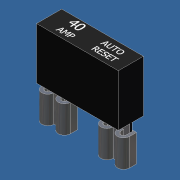
# Autodesk Inventor part: Big CB in Holder
Saved by Autodesk Inventor 2012 (Build 160160000, 160)
## iProperties
Company: Team 801
Created: 2007-09-01
Part Number: Big CB in Holder
Document SubType Name: Modeling
Designer: Jeffrey M
Manufacturer: Standard
Standards Organization: Custom
Mass: 5.35109 g
Surface Area: 29.8147 cm^2
Volume: 5.35109 cm^3
Density: 1 g/cm^3
Catalog Web Link: www.team801.org
Material: Default
PartAngTol0: 0.50 deg
PartAngTol1: 0.50 deg
PartAngTol2: 0.50 deg
PartLinTol0: 0.01 in
PartLinTol1: 0.01 in
PartLinTol2: 0.01 in
PartLinTol3: 0.005 in
PartAngTol3: 0deg30'
Author: Jeffrey M
Autodesk Inventor part; units mm, degrees
ref_plane "YZ Plane (RIGHT)" through (0, 0, 0) normal (1, 0, 0) x (0, 1, 0)
ref_plane "XZ Plane (TOP)" through (0, 0, 0) normal (0, 1, 0) x (-1, 0, 0)
ref_plane "XY Plane (FRONT)" through (0, 0, 0) normal (0, 0, 1) x (1, 0, 0)
sketch "Sketch2" plane through (0, 0, 0) normal (0, 1, 0) x (-1, 0, 0)
  line L0 (-23.1648, 0) -> (17.3736, 0) construction
  line L1 (0, -5.334) -> (0, 7.112) construction
  line L2 (-14.478, 4.445) -> (14.478, 4.445)
  line L3 (14.478, 4.445) -> (14.478, -4.445)
  line L4 (14.478, -4.445) -> (-14.478, -4.445)
  line L5 (-14.478, -4.445) -> (-14.478, 4.445)
  dimension "d0" = 28.956
  dimension "d1" = 8.89
  constraints: 8 end point, 2 parallel, 1 horizontal, 1 perpendicular, 2 other
  measures "d0" distance of L2.start L2.end
  measures "d1" distance of L4.end L2.start
extrude "Extrusion1" add sketch "Sketch2" along normal blind 18.288
sketch "Sketch3" plane through (0, 0, 0) normal (0, -1, 0) x (1, 0, 0)
  line L0 (-14.478, 4.445) -> (-14.478, -4.445) construction
  line L1 (0, 7.112) -> (0, -5.334) construction
  line L2 (-17.3736, 0) -> (23.1648, 0) construction
  line L3 (-14.478, 0.4064) -> (-6.477, 0.4064)
  line L4 (-6.477, 0.4064) -> (-6.477, -0.4064)
  line L5 (-6.477, -0.4064) -> (-14.478, -0.4064)
  line L6 (-14.478, -0.4064) -> (-14.478, 0.4064)
  line L7 (14.478, 0.4064) -> (6.477, 0.4064)
  line L8 (6.477, 0.4064) -> (6.477, -0.4064)
  line L9 (6.477, -0.4064) -> (14.478, -0.4064)
  line L10 (14.478, -0.4064) -> (14.478, 0.4064)
  dimension "d4" = 0.8128
  dimension "d5" = 8.001
  constraints: 16 end point, 4 symmetric about line, 2 parallel, 1 horizontal, 1 perpendicular, 1 point on line, 1 other
  measures "d4" distance between parallel lines of L3 L5
  measures "d5" distance of L4.end L5.end
extrude "Extrusion2" add sketch "Sketch3" along normal blind 12.446
sketch "Sketch4" plane through (0, -12.446, 0) normal (0, -1, 0) x (1, 0, 0)
  line L0 (-6.477, 0.4064) -> (-6.477, -0.4064) projected
  line L1 (-14.478, 0.4064) -> (-6.477, 0.4064) projected
  line L2 (-14.478, -0.4064) -> (-14.478, 0.4064) projected
  line L3 (-6.477, -0.4064) -> (-14.478, -0.4064) projected
  line L4 (-15.5575, -0.9652) -> (-5.3975, -0.9652)
  line L5 (-5.3975, -0.9652) -> (-5.3975, 1.524)
  arc A0 (-5.3975, 1.524) -> (-9.7155, 1.524) centre (-7.5565, 1.524) ccw
  line L6 (-9.7155, 1.524) -> (-11.2395, 1.524)
  arc A1 (-11.2395, 1.524) -> (-15.5575, 1.524) centre (-13.3985, 1.524) ccw
  line L7 (-15.5575, 1.524) -> (-15.5575, -0.9652)
  line L8 (-10.4775, 0.4064) -> (-10.4775, 5.8427) construction
  line L9 (-14.478, 0.4064) -> (-14.478, 1.524)
  arc A2 (-12.319, 1.524) -> (-14.478, 1.524) centre (-13.3985, 1.524) ccw
  line L10 (-12.319, 1.524) -> (-12.319, 0.4064)
  line L11 (-6.477, 0.4064) -> (-6.477, 1.524)
  arc A3 (-6.477, 1.524) -> (-8.636, 1.524) centre (-7.5565, 1.524) ccw
  line L12 (-8.636, 1.524) -> (-8.636, 0.4064)
  point P0 (0, 0)
  dimension "d8" = 0.5588
  dimension "d9" = 10.16
  dimension "d10" = 4.6482
  dimension "d11" = 1.524
  constraints: 18 end point, 8 point on circle, 7 parallel, 6 tangent, 4 centre point, 3 perpendicular, 3 point on line, 2 coincident, 1 midpoint, 1 other
  measures "d8" distance between parallel lines of L4 L3
  measures "d9" distance of L4.start L4.end
  measures "d11" distance of L6.start L6.end
extrude "Extrusion3" add sketch "Sketch4" against normal blind 9.652
mirror "Mirror1" about plane through (0, 0, 0) normal (1, 0, 0) of "Extrusion3"
sketch "Sketch5" plane through (0, 18.288, 0) normal (0, 1, 0) x (1, 0, 0)
  line L0 (-9.1661, 3.7805) -> (-3.0835, 3.7805) construction
  line L1 (-3.0835, 3.7805) -> (-3.0835, -3.7805) construction
  line L2 (-3.0835, -3.7805) -> (-9.1661, -3.7805) construction
  line L3 (-9.1661, -3.7805) -> (-9.1661, 3.7805) construction
  line L4 (2.9146, 2.7245) -> (10.9734, 2.7245) construction
  line L5 (10.9734, 2.7245) -> (10.9734, -2.7322) construction
  line L6 (10.9734, -2.7322) -> (2.9146, -2.7322) construction
  line L7 (2.9146, -2.7322) -> (2.9146, 2.7245) construction
  line L8 (-6.9826, 1.718) -> (-7.3457, 1.718)
  line L9 (-7.3457, 1.718) -> (-7.3457, 0.6707)
  line L10 (-7.3457, 0.6707) -> (-7.7384, 0.6707)
  line L11 (-7.7384, 0.6707) -> (-7.7384, 1.718)
  line L12 (-7.7384, 1.718) -> (-9.0846, 1.718)
  line L13 (-9.0846, 1.718) -> (-9.0846, 2.1478)
  line L14 (-9.0846, 2.1478) -> (-7.7211, 3.7187)
  line L15 (-7.7211, 3.7187) -> (-7.3457, 3.7187)
  line L16 (-7.3457, 3.7187) -> (-7.3457, 2.0465)
  line L17 (-7.3457, 2.0465) -> (-6.9826, 2.0465)
  line L18 (-6.9826, 2.0465) -> (-6.9826, 1.718)
  line L19 (-7.7384, 2.0465) -> (-7.7384, 3.2371)
  line L20 (-7.7384, 3.2371) -> (-8.7635, 2.0465)
  line L21 (-8.7635, 2.0465) -> (-7.7384, 2.0465)
  spline S0 degree 2 poles (-4.7596, 2.1947) (-4.7596, 1.3747) (-5.2363, 0.6065) (-5.7328, 0.6065) knots 0 0 0 1 2 2 2
  spline S1 degree 2 poles (-5.7328, 0.6065) (-6.2367, 0.6065) (-6.7084, 1.3895) (-6.7084, 2.1923) knots 0 0 0 1 2 2 2
  spline S2 degree 2 poles (-6.7084, 2.1923) (-6.7084, 3.0172) (-6.2317, 3.7805) (-5.7328, 3.7805) knots 0 0 0 1 2 2 2
  spline S3 degree 2 poles (-5.7328, 3.7805) (-5.2314, 3.7805) (-4.7596, 2.9901) (-4.7596, 2.1947) knots 0 0 0 1 2 2 2
  spline S4 degree 2 poles (-5.2832, 1.266) (-5.2239, 1.4167) (-5.1745, 1.881) (-5.1745, 2.1947) knots 0 0 0 1 2 2 2
  spline S5 degree 2 poles (-5.1745, 2.1947) (-5.1745, 2.5084) (-5.2239, 2.9703) (-5.2857, 3.1259) knots 0 0 0 1 2 2 2
  spline S6 degree 2 poles (-5.2857, 3.1259) (-5.3474, 3.2815) (-5.5623, 3.4421) (-5.7328, 3.4421) knots 0 0 0 1 2 2 2
  spline S7 degree 2 poles (-5.7328, 3.4421) (-5.9032, 3.4421) (-6.123, 3.2815) (-6.1873, 3.121) knots 0 0 0 1 2 2 2
  spline S8 degree 2 poles (-6.1873, 3.121) (-6.249, 2.9654) (-6.2935, 2.4911) (-6.2935, 2.1923) knots 0 0 0 1 2 2 2
  spline S9 degree 2 poles (-6.2935, 2.1923) (-6.2935, 1.8712) (-6.2539, 1.4414) (-6.1897, 1.2734) knots 0 0 0 1 2 2 2
  spline S10 degree 2 poles (-6.1897, 1.2734) (-6.1304, 1.1153) (-5.9106, 0.9449) (-5.7328, 0.9449) knots 0 0 0 1 2 2 2
  spline S11 degree 2 poles (-5.7328, 0.9449) (-5.5648, 0.9449) (-5.345, 1.1055) (-5.2832, 1.266) knots 0 0 0 1 2 2 2
  line L22 (-9.1793, -3.067) -> (-8.4942, -1.035)
  line L23 (-8.4942, -1.035) -> (-8.1616, -1.035)
  line L24 (-8.1616, -1.035) -> (-7.4766, -3.067)
  line L25 (-7.4766, -3.067) -> (-7.7615, -3.067)
  line L26 (-7.7615, -3.067) -> (-7.9459, -2.4989)
  line L27 (-7.9459, -2.4989) -> (-8.7215, -2.4989)
  line L28 (-8.7215, -2.4989) -> (-8.9059, -3.067)
  line L29 (-8.9059, -3.067) -> (-9.1793, -3.067)
  line L30 (-8.02, -2.2683) -> (-8.3345, -1.3116)
  line L31 (-8.3345, -1.3116) -> (-8.6474, -2.2683)
  line L32 (-8.6474, -2.2683) -> (-8.02, -2.2683)
  line L33 (-5.5418, -3.067) -> (-5.8118, -3.067)
  line L34 (-5.8118, -3.067) -> (-5.8118, -1.3166)
  line L35 (-5.8118, -1.3166) -> (-6.342, -2.5071)
  line L36 (-6.342, -2.5071) -> (-6.5067, -2.5071)
  line L37 (-6.5067, -2.5071) -> (-7.032, -1.3166)
  line L38 (-7.032, -1.3166) -> (-7.032, -3.067)
  line L39 (-7.032, -3.067) -> (-7.2839, -3.067)
  line L40 (-7.2839, -3.067) -> (-7.2839, -1.035)
  line L41 (-7.2839, -1.035) -> (-6.9151, -1.035)
  line L42 (-6.9151, -1.035) -> (-6.4079, -2.1662)
  line L43 (-6.4079, -2.1662) -> (-5.9172, -1.035)
  line L44 (-5.9172, -1.035) -> (-5.5418, -1.035)
  line L45 (-5.5418, -1.035) -> (-5.5418, -3.067)
  spline S12 degree 2 poles (-3.8457, -1.6475) (-3.8457, -1.7793) (-3.9395, -2.0164) (-4.0235, -2.0987) knots 0 0 0 1 2 2 2
  spline S13 degree 2 poles (-4.0235, -2.0987) (-4.1289, -2.2025) (-4.4138, -2.3095) (-4.6311, -2.3095) knots 0 0 0 1 2 2 2
  line L46 (-4.6311, -2.3095) -> (-4.86, -2.3095)
  line L47 (-4.86, -2.3095) -> (-4.86, -3.067)
  line L48 (-4.86, -3.067) -> (-5.1301, -3.067)
  line L49 (-5.1301, -3.067) -> (-5.1301, -1.035)
  line L50 (-5.1301, -1.035) -> (-4.6196, -1.035)
  spline S14 degree 2 poles (-4.6196, -1.035) (-4.4385, -1.035) (-4.1849, -1.0942) (-4.0877, -1.1618) knots 0 0 0 1 2 2 2
  spline S15 degree 2 poles (-4.0877, -1.1618) (-3.9741, -1.2392) (-3.8457, -1.4779) (-3.8457, -1.6475) knots 0 0 0 1 2 2 2
  spline S16 degree 2 poles (-4.1273, -1.6558) (-4.1273, -1.5504) (-4.1997, -1.3956) (-4.2738, -1.3462) knots 0 0 0 1 2 2 2
  spline S17 degree 2 poles (-4.2738, -1.3462) (-4.338, -1.3034) (-4.5093, -1.2688) (-4.6361, -1.2688) knots 0 0 0 1 2 2 2
  line L51 (-4.6361, -1.2688) -> (-4.86, -1.2688)
  line L52 (-4.86, -1.2688) -> (-4.86, -2.079)
  line L53 (-4.86, -2.079) -> (-4.6756, -2.079)
  spline S18 degree 2 poles (-4.6756, -2.079) (-4.5109, -2.079) (-4.3084, -2.0263) (-4.2425, -1.9571) knots 0 0 0 1 2 2 2
  spline S19 degree 2 poles (-4.2425, -1.9571) (-4.1816, -1.8962) (-4.1273, -1.7529) (-4.1273, -1.6558) knots 0 0 0 1 2 2 2
  line L54 (2.9014, 0.6497) -> (3.5864, 2.6817)
  line L55 (3.5864, 2.6817) -> (3.919, 2.6817)
  line L56 (3.919, 2.6817) -> (4.6041, 0.6497)
  line L57 (4.6041, 0.6497) -> (4.3192, 0.6497)
  line L58 (4.3192, 0.6497) -> (4.1348, 1.2178)
  line L59 (4.1348, 1.2178) -> (3.3592, 1.2178)
  line L60 (3.3592, 1.2178) -> (3.1747, 0.6497)
  line L61 (3.1747, 0.6497) -> (2.9014, 0.6497)
  line L62 (4.0607, 1.4483) -> (3.7461, 2.405)
  line L63 (3.7461, 2.405) -> (3.4333, 1.4483)
  line L64 (3.4333, 1.4483) -> (4.0607, 1.4483)
  spline S20 degree 2 poles (5.5064, 0.6069) (5.3269, 0.6069) (5.0602, 0.7007) (4.9663, 0.7946) knots 0 0 0 1 2 2 2
  spline S21 degree 2 poles (4.9663, 0.7946) (4.8593, 0.9) (4.772, 1.1964) (4.772, 1.4137) knots 0 0 0 1 2 2 2
  line L65 (4.772, 1.4137) -> (4.772, 2.6817)
  line L66 (4.772, 2.6817) -> (5.0421, 2.6817)
  line L67 (5.0421, 2.6817) -> (5.0421, 1.4137)
  spline S22 degree 2 poles (5.0421, 1.4137) (5.0421, 1.2721) (5.0783, 1.0811) (5.1293, 1.0037) knots 0 0 0 1 2 2 2
  spline S23 degree 2 poles (5.1293, 1.0037) (5.1837, 0.9214) (5.3714, 0.8374) (5.5064, 0.8374) knots 0 0 0 1 2 2 2
  spline S24 degree 2 poles (5.5064, 0.8374) (5.6332, 0.8374) (5.8308, 0.9214) (5.8852, 1.0037) knots 0 0 0 1 2 2 2
  spline S25 degree 2 poles (5.8852, 1.0037) (5.9362, 1.0811) (5.9724, 1.2705) (5.9724, 1.4071) knots 0 0 0 1 2 2 2
  line L68 (5.9724, 1.4071) -> (5.9724, 2.6817)
  line L69 (5.9724, 2.6817) -> (6.2425, 2.6817)
  line L70 (6.2425, 2.6817) -> (6.2425, 1.4137)
  spline S26 degree 2 poles (6.2425, 1.4137) (6.2425, 1.2013) (6.1569, 0.8983) (6.0482, 0.7946) knots 0 0 0 1 2 2 2
  spline S27 degree 2 poles (6.0482, 0.7946) (5.951, 0.6991) (5.6942, 0.6069) (5.5064, 0.6069) knots 0 0 0 1 2 2 2
  line L71 (7.1037, 0.6497) -> (7.1037, 2.4413)
  line L72 (7.1037, 2.4413) -> (6.422, 2.4413)
  line L73 (6.422, 2.4413) -> (6.422, 2.6817)
  line L74 (6.422, 2.6817) -> (8.0555, 2.6817)
  line L75 (8.0555, 2.6817) -> (8.0555, 2.4413)
  line L76 (8.0555, 2.4413) -> (7.3738, 2.4413)
  line L77 (7.3738, 2.4413) -> (7.3738, 0.6497)
  line L78 (7.3738, 0.6497) -> (7.1037, 0.6497)
  spline S28 degree 2 poles (9.6989, 2.4495) (9.8141, 2.3145) (9.9426, 1.9193) (9.9426, 1.6657) knots 0 0 0 1 2 2 2
  spline S29 degree 2 poles (9.9426, 1.6657) (9.9426, 1.4187) (9.8174, 1.0185) (9.6989, 0.8835) knots 0 0 0 1 2 2 2
  spline S30 degree 2 poles (9.6989, 0.8835) (9.5737, 0.7419) (9.2427, 0.6069) (9.0435, 0.6069) knots 0 0 0 1 2 2 2
  spline S31 degree 2 poles (9.0435, 0.6069) (8.8377, 0.6069) (8.5083, 0.7468) (8.3881, 0.8835) knots 0 0 0 1 2 2 2
  spline S32 degree 2 poles (8.3881, 0.8835) (8.2712, 1.0185) (8.1461, 1.4154) (8.1461, 1.6657) knots 0 0 0 1 2 2 2
  spline S33 degree 2 poles (8.1461, 1.6657) (8.1461, 1.9209) (8.2729, 2.3095) (8.3898, 2.4495) knots 0 0 0 1 2 2 2
  spline S34 degree 2 poles (8.3898, 2.4495) (8.5083, 2.5845) (8.8393, 2.7245) (9.0435, 2.7245) knots 0 0 0 1 2 2 2
  spline S35 degree 2 poles (9.0435, 2.7245) (9.251, 2.7245) (9.5836, 2.5796) (9.6989, 2.4495) knots 0 0 0 1 2 2 2
  spline S36 degree 2 poles (9.661, 1.6657) (9.661, 1.8666) (9.5737, 2.1778) (9.4947, 2.2799) knots 0 0 0 1 2 2 2
  spline S37 degree 2 poles (9.4947, 2.2799) (9.414, 2.3853) (9.1868, 2.4907) (9.0451, 2.4907) knots 0 0 0 1 2 2 2
  spline S38 degree 2 poles (9.0451, 2.4907) (8.8986, 2.4907) (8.6779, 2.3886) (8.594, 2.2799) knots 0 0 0 1 2 2 2
  spline S39 degree 2 poles (8.594, 2.2799) (8.5133, 2.1761) (8.4276, 1.8633) (8.4276, 1.6657) knots 0 0 0 1 2 2 2
  spline S40 degree 2 poles (8.4276, 1.6657) (8.4276, 1.2655) (8.7636, 0.8407) (9.0451, 0.8407) knots 0 0 0 1 2 2 2
  spline S41 degree 2 poles (9.0451, 0.8407) (9.3267, 0.8407) (9.661, 1.2655) (9.661, 1.6657) knots 0 0 0 1 2 2 2
  line L79 (4.693, -2.696) -> (4.3422, -2.696)
  line L80 (4.3422, -2.696) -> (3.7, -1.8874)
  line L81 (3.7, -1.8874) -> (3.3905, -1.8874)
  line L82 (3.3905, -1.8874) -> (3.3905, -2.696)
  line L83 (3.3905, -2.696) -> (3.1204, -2.696)
  line L84 (3.1204, -2.696) -> (3.1204, -0.664)
  line L85 (3.1204, -0.664) -> (3.644, -0.664)
  spline S42 degree 2 poles (3.644, -0.664) (3.8186, -0.664) (4.0541, -0.7018) (4.1611, -0.771) knots 0 0 0 1 2 2 2
  spline S43 degree 2 poles (4.1611, -0.771) (4.2681, -0.8402) (4.3916, -1.0559) (4.3916, -1.2156) knots 0 0 0 1 2 2 2
  spline S44 degree 2 poles (4.3916, -1.2156) (4.3916, -1.4379) (4.1644, -1.7392) (3.9701, -1.8117) knots 0 0 0 1 2 2 2
  line L86 (3.9701, -1.8117) -> (4.693, -2.696)
  spline S45 degree 2 poles (4.1101, -1.237) (4.1101, -1.1481) (4.0475, -1.0114) (3.9816, -0.967) knots 0 0 0 1 2 2 2
  spline S46 degree 2 poles (3.9816, -0.967) (3.924, -0.9291) (3.7708, -0.8978) (3.6589, -0.8978) knots 0 0 0 1 2 2 2
  line L87 (3.6589, -0.8978) -> (3.3905, -0.8978)
  line L88 (3.3905, -0.8978) -> (3.3905, -1.6619)
  line L89 (3.3905, -1.6619) -> (3.6276, -1.6619)
  spline S47 degree 2 poles (3.6276, -1.6619) (3.7445, -1.6619) (3.9306, -1.6207) (3.9948, -1.5565) knots 0 0 0 1 2 2 2
  spline S48 degree 2 poles (3.9948, -1.5565) (4.0541, -1.5005) (4.1101, -1.3424) (4.1101, -1.237) knots 0 0 0 1 2 2 2
  line L90 (4.8543, -2.696) -> (4.8543, -0.664)
  line L91 (4.8543, -0.664) -> (6.1256, -0.664)
  line L92 (6.1256, -0.664) -> (6.1256, -0.9044)
  line L93 (6.1256, -0.9044) -> (5.1244, -0.9044)
  line L94 (5.1244, -0.9044) -> (5.1244, -1.461)
  line L95 (5.1244, -1.461) -> (6.0581, -1.461)
  line L96 (6.0581, -1.461) -> (6.0581, -1.7014)
  line L97 (6.0581, -1.7014) -> (5.1244, -1.7014)
  line L98 (5.1244, -1.7014) -> (5.1244, -2.4555)
  line L99 (5.1244, -2.4555) -> (6.1256, -2.4555)
  line L100 (6.1256, -2.4555) -> (6.1256, -2.696)
  line L101 (6.1256, -2.696) -> (4.8543, -2.696)
  spline S49 degree 2 poles (6.9884, -2.7322) (6.7678, -2.7322) (6.4582, -2.64) (6.3215, -2.5741) knots 0 0 0 1 2 2 2
  line L102 (6.3215, -2.5741) -> (6.3215, -2.2349)
  line L103 (6.3215, -2.2349) -> (6.3413, -2.2349)
  spline S50 degree 2 poles (6.3413, -2.2349) (6.4747, -2.36) (6.8122, -2.4984) (6.9687, -2.4984) knots 0 0 0 1 2 2 2
  spline S51 degree 2 poles (6.9687, -2.4984) (7.1926, -2.4984) (7.4215, -2.3123) (7.4215, -2.1591) knots 0 0 0 1 2 2 2
  spline S52 degree 2 poles (7.4215, -2.1591) (7.4215, -2.0373) (7.3013, -1.8858) (7.1712, -1.8479) knots 0 0 0 1 2 2 2
  spline S53 degree 2 poles (7.1712, -1.8479) (7.0774, -1.8216) (6.9209, -1.7854) (6.804, -1.7557) knots 0 0 0 1 2 2 2
  spline S54 degree 2 poles (6.804, -1.7557) (6.6986, -1.7277) (6.5323, -1.6437) (6.4681, -1.5762) knots 0 0 0 1 2 2 2
  spline S55 degree 2 poles (6.4681, -1.5762) (6.4055, -1.5087) (6.3364, -1.3276) (6.3364, -1.209) knots 0 0 0 1 2 2 2
  spline S56 degree 2 poles (6.3364, -1.209) (6.3364, -0.962) (6.7217, -0.6277) (7.0197, -0.6277) knots 0 0 0 1 2 2 2
  spline S57 degree 2 poles (7.0197, -0.6277) (7.191, -0.6277) (7.494, -0.6953) (7.6241, -0.7595) knots 0 0 0 1 2 2 2
  line L104 (7.6241, -0.7595) -> (7.6241, -1.0822)
  line L105 (7.6241, -1.0822) -> (7.6043, -1.0822)
  spline S58 degree 2 poles (7.6043, -1.0822) (7.5071, -0.9933) (7.2042, -0.8616) (7.0378, -0.8616) knots 0 0 0 1 2 2 2
  spline S59 degree 2 poles (7.0378, -0.8616) (6.8501, -0.8616) (6.6179, -1.0378) (6.6179, -1.181) knots 0 0 0 1 2 2 2
  spline S60 degree 2 poles (6.6179, -1.181) (6.6179, -1.3095) (6.7546, -1.4626) (6.8831, -1.4972) knots 0 0 0 1 2 2 2
  spline S61 degree 2 poles (6.8831, -1.4972) (6.9687, -1.5202) (7.2173, -1.5795) (7.2997, -1.6042) knots 0 0 0 1 2 2 2
  spline S62 degree 2 poles (7.2997, -1.6042) (7.5088, -1.6684) (7.7031, -1.927) (7.7031, -2.1163) knots 0 0 0 1 2 2 2
  spline S63 degree 2 poles (7.7031, -2.1163) (7.7031, -2.2365) (7.6059, -2.4671) (7.5187, -2.5478) knots 0 0 0 1 2 2 2
  spline S64 degree 2 poles (7.5187, -2.5478) (7.4215, -2.6367) (7.1745, -2.7322) (6.9884, -2.7322) knots 0 0 0 1 2 2 2
  line L106 (7.9781, -2.696) -> (7.9781, -0.664)
  line L107 (7.9781, -0.664) -> (9.2493, -0.664)
  line L108 (9.2493, -0.664) -> (9.2493, -0.9044)
  line L109 (9.2493, -0.9044) -> (8.2482, -0.9044)
  line L110 (8.2482, -0.9044) -> (8.2482, -1.461)
  line L111 (8.2482, -1.461) -> (9.1818, -1.461)
  line L112 (9.1818, -1.461) -> (9.1818, -1.7014)
  line L113 (9.1818, -1.7014) -> (8.2482, -1.7014)
  line L114 (8.2482, -1.7014) -> (8.2482, -2.4555)
  line L115 (8.2482, -2.4555) -> (9.2493, -2.4555)
  line L116 (9.2493, -2.4555) -> (9.2493, -2.696)
  line L117 (9.2493, -2.696) -> (7.9781, -2.696)
  line L118 (10.02, -2.696) -> (10.02, -0.9044)
  line L119 (10.02, -0.9044) -> (9.3383, -0.9044)
  line L120 (9.3383, -0.9044) -> (9.3383, -0.664)
  line L121 (9.3383, -0.664) -> (10.9718, -0.664)
  line L122 (10.9718, -0.664) -> (10.9718, -0.9044)
  line L123 (10.9718, -0.9044) -> (10.29, -0.9044)
  line L124 (10.29, -0.9044) -> (10.29, -2.696)
  line L125 (10.29, -2.696) -> (10.02, -2.696)
  dimension "d1" = 8.89
  constraints: 4 other
extrude "Extrusion4" cut sketch "Sketch5" against normal blind 0.0025
body "Solid1"
